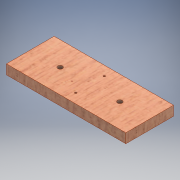
# Autodesk Inventor part: extremite
Saved by Autodesk Inventor 2017 SP1 (Build 210196100, 196)
## iProperties
Created: 2017-10-26
Part Number: extremite
Material: Wood (Oak)
Document SubType Name: Modeling
Designer: Biscuit
Density: 0.76 g/cm^3
Appearance: White Oak - Natural Medium Gloss
Mass: 37.8508 g
Surface Area: 131.571 cm^2
Volume: 49.8037 cm^3
Author: Biscuit
Autodesk Inventor part; units mm, degrees
ref_plane "YZ Plane" through (0, 0, 0) normal (1, 0, 0) x (0, 1, 0)
ref_plane "XZ Plane" through (0, 0, 0) normal (0, 1, 0) x (-1, 0, 0)
ref_plane "XY Plane" through (0, 0, 0) normal (0, 0, 1) x (1, 0, 0)
sketch "Sketch1" plane through (0, 0, 0) normal (0, 0, 1) x (1, 0, 0)
  line L0 (0, 0) -> (125, 0)
  line L1 (125, 0) -> (125, 50)
  line L2 (125, 50) -> (0, 50)
  line L3 (0, 50) -> (0, 0)
  dimension "d0" = 125
  dimension "d1" = 50
  constraints: 8 end point, 2 parallel, 1 horizontal, 1 perpendicular
  measures "d0" distance of L1.end L2.end
  measures "d1" distance of L0.end L1.end
extrude "Extrusion1" add sketch "Sketch1" along normal blind 10
sketch "Sketch2" plane through (0, 0, 10) normal (0, 0, 1) x (1, 0, 0)
  circle A0 centre (31.25, 25) radius 2.5
  circle A1 centre (93.75, 25) radius 2.5
  line L0 (125, 50) -> (0, 50) projected
  line L1 (0, 0) -> (125, 0) projected
  line L2 (125, 0) -> (125, 50) projected
  line L3 (0, 50) -> (0, 0) projected
  dimension "d4" = 5
  dimension "d5" = 5
  dimension "d6" = 62.5
  dimension "d7" = 25
  dimension "d8" = 50
  dimension "d9" = 125
  dimension "d10" = 31.25
  dimension "d26" = 25
  dimension "d27" = 31.25
  constraints: 2 centre point
  measures "d4" diameter of A0
  measures "d5" diameter of A1
  measures "d6" distance of A1.centre A0.centre
  measures "d7" distance from line of L0 A1.centre
  measures "d8" distance between parallel lines of L1 L0
  measures "d9" distance between parallel lines of L2 L3
  measures "d10" distance from line of L2 A1.centre
  measures "d26" distance from line of L1 A0.centre
  measures "d27" distance from line of L3 A0.centre
extrude "Extrusion2" cut sketch "Sketch2" against normal blind 5 contours A0 | A1
sketch "Sketch3" plane through (0, 0, 10) normal (0, 0, 1) x (1, 0, 0)
  circle A0 centre (62.5, 40) radius 1
  circle A1 centre (62.5, 10) radius 1
  line L0 (0, 0) -> (125, 0) projected
  line L1 (125, 50) -> (0, 50) projected
  line L2 (125, 0) -> (125, 50) projected
  line L3 (0, 50) -> (0, 0) projected
  dimension "d13" = 2
  dimension "d14" = 2
  dimension "d16" = 50
  dimension "d17" = 10
  dimension "d20" = 125
  dimension "d23" = 62.5
  dimension "d24" = 62.5
  dimension "d25" = 30
  constraints: 2 centre point
  measures "d13" diameter of A0
  measures "d14" diameter of A1
  measures "d16" distance between parallel lines of L0 L1
  measures "d17" distance from line of L0 A1.centre
  measures "d20" distance between parallel lines of L3 L2
  measures "d23" distance from line of L2 A0.centre
  measures "d24" distance from line of L2 A1.centre
  measures "d25" distance of A0.centre A1.centre
extrude "Extrusion3" cut sketch "Sketch3" against normal blind 10 contours A0 | A1
equation "\"d7\" = 0.5 * d8"
equation "\"d10\" = 0.5 * d9 - 0.5 * d6"
equation "\"d26\" = d7"
equation "\"d17\" = 0.5 * d16 - 0.5 * d25"
equation "\"d23\" = 0.5 * d20"
equation "\"d24\" = d23"
equation "\"d15\" = 0.5 * d16"
body "Solid1"
